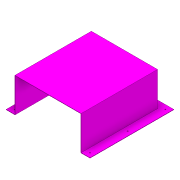
# Autodesk Inventor part: SidePanelCover
Saved by Autodesk Inventor 2017 (Build 210142000, 142)
## iProperties
Created: 2017-10-03
Part Number: SidePanelCover
Material: Generic
Document SubType Name: Modeling
Designer: Kathryn Rosie
Density: 1 g/cm^3
Appearance: Default
Author: Kathryn Rosie
Autodesk Inventor part; units mm, degrees
ref_plane "YZ Plane" through (0, 0, 0) normal (1, 0, 0) x (0, 1, 0)
ref_plane "XZ Plane" through (0, 0, 0) normal (0, 1, 0) x (-1, 0, 0)
ref_plane "XY Plane" through (0, 0, 0) normal (0, 0, 1) x (1, 0, 0)
sketch "Sketch1" plane through (0, 0, 0) normal (0, 0, 1) x (1, 0, 0)
  line L0 (-247, -247) -> (247, -247)
  line L1 (247, -247) -> (247, 247)
  line L2 (247, 247) -> (-247, 247)
  line L3 (-247, 247) -> (-247, -247)
  line L4 (-247, -247) -> (247, 247) construction
  line L5 (247, -247) -> (-247, 247) construction
  line L6 (-195, -247) -> (-195, 203)
  line L7 (-195, 203) -> (195, 203)
  line L8 (195, 203) -> (195, -247)
  line L9 (195, -247) -> (-195, -247)
  line L10 (0, 247) -> (0, -247) construction
  point P0 (0, 0)
  dimension "d0" = 494
  dimension "d1" = 494
  dimension "d4" = 390
  dimension "d5" = 450
  constraints: 22 end point, 4 midpoint, 3 parallel, 2 horizontal, 2 point on line, 1 collinear, 1 perpendicular, 1 vertical, 1 other
  measures "d0" distance of L0.start L0.end
  measures "d1" distance of L1.end L0.end
  measures "d4" distance of L6.end L7.end
  measures "d5" distance of L7.end L8.end
extrude "Extrusion2" add sketch "Sketch1" along normal blind 200 contours L6 L7 L8 L0
shell "Shell2" thickness 2 removed faces 1 at (65, -97, 0)
extrude "Extrusion3" add sketch "Sketch1" against normal blind 2 contours L3 L2 L1 L0 L8 L7 L6
hole "Hole1" at (-222, 222, 0) direction (0, 0, -1) diameter 6 end through all
pattern_linear "Rectangular Pattern1" count 3 spacing 222 along (1, 0, 0) count 3 spacing 222 along (0, -1, 0) of "Hole1"
sketch "Sketch2" plane through (-193, -245, 0) normal (0, 1, 0) x (1, 0, 0)
  line L0 (0, 0) -> (386, 0) projected
  line L1 (0, 0) -> (0, -198) projected
  line L2 (0, -198) -> (386, -198) projected
  line L3 (386, 0) -> (386, -198) projected
  point P0 (193, 0)
extrude "Extrusion4" cut sketch "Sketch2" against normal up to next
body "Solid1"
